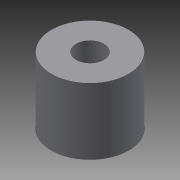
# Autodesk Inventor part: Стойка_1
Saved by Autodesk Inventor 2014 (Build 180170000, 170)
## iProperties
Created: 2017-02-08
Part Number: Стойка_1
Material: Типовые
Document SubType Name: Modeling
Designer: Nikopol
Density: 1 g/cm^3
Appearance: По умолчанию
Author: Nikopol
Autodesk Inventor part; units mm, degrees
ref_plane "YZ Plane" through (0, 0, 0) normal (1, 0, 0) x (0, 1, 0)
ref_plane "XZ Plane" through (0, 0, 0) normal (0, 1, 0) x (-1, 0, 0)
ref_plane "XY Plane" through (0, 0, 0) normal (0, 0, 1) x (1, 0, 0)
sketch "Эскиз1" plane through (0, 0, 0) normal (0, 0, 1) x (1, 0, 0)
  circle A0 centre (0, 0) radius 1.25
  circle A1 centre (0, 0) radius 3.5
  dimension "d0" = 2.5
  dimension "d1" = 7
  constraints: 2 centre point, 2 coincident
  measures "d0" diameter of A0
  measures "d1" diameter of A1
extrude "Выдавливание1" add sketch "Эскиз1" along normal blind 6
